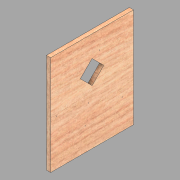
# Autodesk Inventor part: x_axis_wood_mount
Saved by Autodesk Inventor 2020 (Build 240168000, 168)
## iProperties
Created: 2021-04-20
Part Number: x_axis_wood_mount
Material: Wood (Birch)
Document SubType Name: Modeling
Designer: griss
Density: 0.55 g/cm^3
Appearance: Birch - Natural Polished
Author: griss
Autodesk Inventor part; units mm, degrees
ref_plane "YZ Plane" through (0, 0, 0) normal (1, 0, 0) x (0, 1, 0)
ref_plane "XZ Plane" through (0, 0, 0) normal (0, 1, 0) x (-1, 0, 0)
ref_plane "XY Plane" through (0, 0, 0) normal (0, 0, 1) x (1, 0, 0)
sketch "Sketch1" plane through (0, 0, 0) normal (0, 0, 1) x (1, 0, 0)
  line L0 (-3.175, 76.2) -> (3.175, 76.2)
  line L1 (3.175, 76.2) -> (3.175, -76.2)
  line L2 (3.175, -76.2) -> (-3.175, -76.2)
  line L3 (-3.175, -76.2) -> (-3.175, 76.2)
  line L4 (-3.175, 76.2) -> (3.175, -76.2) construction
  line L5 (3.175, 76.2) -> (-3.175, -76.2) construction
  point P0 (0, 0)
  dimension "d0" = 6.35
  dimension "d1" = 152.4
  constraints: 12 end point, 2 midpoint, 2 parallel, 1 horizontal, 1 perpendicular
  measures "d0" distance of L1.end L2.end
  measures "d1" distance of L0.end L1.end
extrude "Extrusion1" add sketch "Sketch1" along normal mid plane 127
sketch "Sketch2" plane through (3.175, -76.2, 63.5) normal (1, 0, 0) x (0, 0, -1)
  line L0 (63.5, 83.6395) -> (81.4605, 101.6)
  line L1 (81.4605, 101.6) -> (63.5, 119.5605)
  line L2 (63.5, 119.5605) -> (45.5395, 101.6)
  line L3 (45.5395, 101.6) -> (63.5, 83.6395)
  line L4 (63.5, 83.6395) -> (63.5, 119.5605) construction
  line L5 (81.4605, 101.6) -> (45.5395, 101.6) construction
  line L6 (63.5, 83.6395) -> (88.9, 83.6395) construction
  line L7 (127, 152.4) -> (0, 152.4) projected
  point P0 (63.5, 76.2)
  point P1 (63.5, 101.6)
  point P2 (63.5, 152.4)
  point P3 (63.5, 101.6)
  dimension "d4" = 25.4
  dimension "d5" = 45
  dimension "d6" = 25.4
  dimension "d7" = 50.8
  constraints: 14 end point, 4 midpoint, 2 parallel, 1 equal length, 1 horizontal, 1 perpendicular, 1 vertical alignment
  measures "d4" distance of L0.start L0.end
  measures "d5" angle of L6 L0
  measures "d6" distance of L1.end L0.end
  measures "d7" distance from line of point (63.5, 101.6) L7
extrude "Extrusion2" cut sketch "Sketch2" against normal up to surface (6.35 mm away)
body "Solid1"
